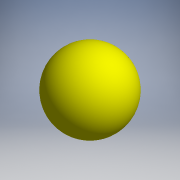
# Autodesk Inventor part: SKF_624-2Z_PART3
Saved by Autodesk Inventor 2017.3 (Build 213256000, 256)
## iProperties
Part Number: SKF_624-2Z_PART3
Material: Generic
Catalog Web Link: www.cadenas.de
Description: -Deep groove ball bearings
Vendor: SKF
Document SubType Name: Modeling
Designer: partserver
Manufacturer: SKF
Mass: 3 g
Surface Area: 0.178102 cm^2
Volume: 0.00706768 cm^3
Density: 1 g/cm^3
Appearance: PSOLRGB-192-192-192
Category: PARTsolutions
Company: SKF
Title: SKF_624-2Z_PART3
Author: Cadenas PARTsolutions
Comments: Deep groove ball bearings
PSOL_IDENT_0: {$CADENAS_DATA\23d-libs\skf\bearings_units_and_housings\ball_bearings\deep_groove_ball_bearings\bb1_
PSOL_IDENT_1: 001_101.prj},199 {VTYP=3D},{NB=SKF_624-2Z_PART3},{LINA=SKF_624-2Z_PART3},{NN=BB1_001_101_PART3},{NOP
PSOL_IDENT_2: RJ=TRUE},{DATE=11.06.2021 05:15:49},{GEOMDATE=07.06.2021 05:44:42},{VERSION=},{LINEID=11560},{WBVAR=
PSOL_IDENT_3: },{WBNUMERIC=}  {NB=SKF_624-2Z_PART3},{LINA=SKF_624-2Z_PART3},{KT=DUMMY},{DESIGNATION=624-2Z},{R12=0
PSOL_IDENT_4: .20},{DD=4.000},{D=13.000},{B=5.000},{C=},{CX=},{CXX=},{CA=0.000},{XXVARIANT=},{XXDESIGN=Single row}
PSOL_IDENT_5: ,{XXSEALING=Shield on both sides},{DESIGN=dgbbz},{DESIGNIR=dgbbz},{VARIANT=},{DD1=6.95},{DD2=},{DD2X=
PSOL_IDENT_6: },{DD2A=0.00},{D1=10.30},{D1X=MIN},{D2=11.2},{D2A=11.20},{D3=},{D3X=},{D3A=0.000},{D4=},{HH=MIN},{BB=
PSOL_IDENT_7: MIN},{BBX=},{BBA=0.000},{FF=},{R0MAX=MIN},{R0=MIN},{PITCH=8.70},{DW=2.381},{DDAMIN=5.800},{DDAMAX=6.
PSOL_IDENT_8: 600},{DDBMIN=MIN},{DDBMAX=MIN},{DBMIN=MIN},{DAMAX=11.200},{BBAMIN=MIN},{CAMAX=MIN},{RAMAX=0.200},{LO
PSOL_IDENT_9: AD1=0.936},{LOAD2=0.290},{LOAD3=0.012},{SPEED1=110000},{SPEED2=53000},{KR=0.025},{F0=7.300},{Z=7},{I
PSOL_IDENT_10: I=1},{MASS=0.003},{BEARING=624-2Z},{RING=},{HELP=1.350},{HELP2=0.900},{DD1ALG=3.475},{YALG=3.475},{P
PSOL_IDENT_11: ITCH1=8.700},{DW1=2.381},{YALG1=5.150},{HALG1=1.350},{SH=3.475},{CU=0.524},{HALG=1.475},{B1=0},{SHIE
PSOL_IDENT_12: LDHELP=2},{D4A=0.000},{FFA=0.000},{RS1=}
NB: SKF_624-2Z_PART3
NT: Deep groove ball bearings
NBSYN: SKF_$DESIGNATION._PART3
LINA: SKF_624-2Z_PART3
CATALOG: SKF
DESIGNATION: 624-2Z
R12: 0.2
DD: 4
D: 13
B: 5
D2: 11.2
LOAD1: 0.936
LOAD2: 0.29
LOAD3: 0.012
SPEED1: 110000
SPEED2: 53000
BEARING: 624-2Z
SUPPLIER: SKF
ARTICLENO: SKF_624-2Z_PART3
BOMINFO: SKF_624-2Z_PART3
CREATOR: CADENAS GmbH
Autodesk Inventor part; units mm, degrees
ref_plane "YZ Plane" through (0, 0, 0) normal (1, 0, 0) x (0, 1, 0)
ref_plane "XZ Plane" through (0, 0, 0) normal (0, 1, 0) x (-1, 0, 0)
ref_plane "XY Plane" through (0, 0, 0) normal (0, 0, 1) x (1, 0, 0)
sketch "Sketch_6" plane through (0, 0, 0) normal (0, 0, 1) x (1, 0, 0)
  line L0 (3.6905, 4.35) -> (1.3095, 4.35)
  arc A0 (3.6905, 4.35) -> (1.3095, 4.35) centre (2.5, 4.35) ccw
  line L1 (3.6905, 4.35) -> (1.3095, 4.35)
  dimension "d0" = 360
  constraints: 4 end point, 2 point on circle, 1 centre point
revolve "Revolution1" add sketch "Sketch_6" angle 360 about axis through (3.6905, 4.35, 0) along (1, 0, 0)
body "Solid1"
